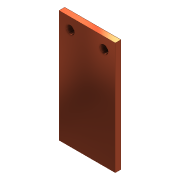
# Autodesk Inventor part: Placa PCB 40x20
Saved by Autodesk Inventor 2020 (Build 240168000, 168)
## iProperties
Created: 2020-08-13
Part Number: Placa PCB 40x20
Material: Generic
Document SubType Name: Modeling
Designer: Dante
Density: 1 g/cm^3
Appearance: Copper - Polished
Author: Dante
Autodesk Inventor part; units mm, degrees
ref_plane "YZ Plane" through (0, 0, 0) normal (1, 0, 0) x (0, 1, 0)
ref_plane "XZ Plane" through (0, 0, 0) normal (0, 1, 0) x (-1, 0, 0)
ref_plane "XY Plane" through (0, 0, 0) normal (0, 0, 1) x (1, 0, 0)
sketch "Sketch1" plane through (0, 0, 0) normal (0, 0, 1) x (1, 0, 0)
  line L0 (-28.6909, 41.0213) -> (-8.6909, 41.0213)
  line L1 (-8.6909, 41.0213) -> (-8.6909, 1.0213)
  line L2 (-8.6909, 1.0213) -> (-28.6909, 1.0213)
  line L3 (-28.6909, 1.0213) -> (-28.6909, 41.0213)
  circle A0 centre (-24.6909, 37.0213) radius 1.5
  circle A1 centre (-12.6909, 37.0213) radius 1.5
  dimension "d0" = 20
  dimension "d1" = 40
  dimension "d4" = 3
  dimension "d5" = 3
  dimension "d7" = 4
  dimension "d8" = 4
  dimension "d9" = 4
  dimension "d10" = 4
  constraints: 8 end point, 2 centre point, 2 parallel, 1 horizontal, 1 perpendicular
  measures "d0" distance of L1.end L2.end
  measures "d1" distance of L0.end L1.end
  measures "d4" diameter of A0
  measures "d5" diameter of A1
  measures "d7" distance from line of L3 A0.centre
  measures "d8" distance from line of A0.centre L0
  measures "d9" distance from line of A1.centre L1
  measures "d10" distance from line of L0 A1.centre
extrude "Extrusion1" add sketch "Sketch1" along normal blind 2
equation "\"d4\" = d5"
equation "\"d7\" = d9"
equation "\"d8\" = d10"
body "Solid1"
